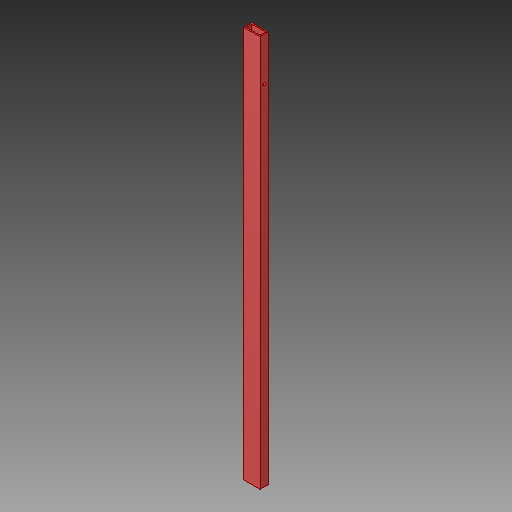
# Autodesk Inventor part: InnerTube
Saved by Autodesk Inventor 2017 (Build 210142000, 142)
## iProperties
Created: 2016-01-26
Part Number: InnerTube
Material: Aluminum 6061
Document SubType Name: Modeling
Designer: steele
Density: 2.7 g/cm^3
Appearance: Smooth - Red
Mass: 840.113 g
Surface Area: 1967.74 cm^2
Volume: 311.153 cm^3
Author: steele
Autodesk Inventor part; units mm, degrees
ref_plane "YZ Plane" through (0, 0, 0) normal (1, 0, 0) x (0, 1, 0)
ref_plane "XZ Plane" through (0, 0, 0) normal (0, 1, 0) x (-1, 0, 0)
ref_plane "XY Plane" through (0, 0, 0) normal (0, 0, 1) x (1, 0, 0)
sketch "Sketch5" plane through (0, 0, 0) normal (0, 1, 0) x (-1, 0, 0)
  line L0 (19.05, 9.525) -> (-19.05, 9.525)
  line L1 (-19.05, 9.525) -> (-19.05, -9.525)
  line L2 (-19.05, -9.525) -> (19.05, -9.525)
  line L3 (19.05, -9.525) -> (19.05, 9.525)
  line L4 (19.05, 9.525) -> (-19.05, -9.525) construction
  line L5 (-19.05, 9.525) -> (19.05, -9.525) construction
  line L6 (15.875, 6.35) -> (-15.875, 6.35)
  line L7 (-15.875, 6.35) -> (-15.875, -6.35)
  line L8 (-15.875, -6.35) -> (15.875, -6.35)
  line L9 (15.875, -6.35) -> (15.875, 6.35)
  line L10 (15.875, 6.35) -> (-15.875, -6.35) construction
  line L11 (-15.875, 6.35) -> (15.875, -6.35) construction
  point P0 (0, 0)
  dimension "d11" = 19.05
  dimension "d12" = 38.1
  dimension "d13" = 3.175
  dimension "d14" = 3.175
  constraints: 24 end point, 4 midpoint, 4 parallel, 2 horizontal, 2 perpendicular
  measures "d11" distance of L2.end L0.start
  measures "d12" distance of L0.start L0.end
  measures "d13" distance between parallel lines of L6 L0
  measures "d14" distance between parallel lines of L3 L9
extrude "Extrusion4" add sketch "Sketch5" along normal blind 923.29
sketch "Sketch6" plane through (-19.05, 0, 9.525) normal (-1, 0, 0) x (0, 0, 1)
  circle A0 centre (-9.525, 821.69) radius 3.175
  line L0 (-19.05, 923.29) -> (0, 923.29) projected
  point P0 (-9.525, 0)
  dimension "d17" = 6.35
  dimension "d18" = 101.6
  constraints: 1 centre point
  measures "d17" diameter of A0
  measures "d18" distance from line of A0.centre L0
extrude "Extrusion6" cut sketch "Sketch6" against normal through all
equation "\"d11\" = tubeWidth"
equation "\"d12\" = tubeBreadth"
equation "\"d13\" = tubeMaterialThickness"
equation "\"d14\" = tubeMaterialThickness"
equation "\"d15\" = tubeLength"
equation "\"d17\" = endOfTravelPostDiam"
equation "\"d18\" = endOfTravellDistanceFromBottom"
equation "\"tubeBreadth\" = 38.1"
equation "\"tubeMaterialThickness\" = 3.175"
equation "\"tubeLength\" = 923.29"
equation "\"tubeWidth\" = 19.05"
equation "\"endOfTravelPostDiam\" = 6.35"
equation "\"endOfTravellDistanceFromBottom\" = 101.6"
body "Solid2"
